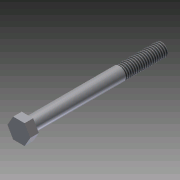
# Autodesk Inventor part: Bolt 1764
Saved by Autodesk Inventor 2011 (Build 150239000, 239)
## iProperties
Created: 2010-02-11
Part Number: Bolt 1764
Document SubType Name: Modeling
Designer: jrobinson
Density: 1 g/cm^3
Author: jrobinson
Autodesk Inventor part; units mm, degrees
ref_plane "YZ Plane" through (0, 0, 0) normal (1, 0, 0) x (0, 1, 0)
ref_plane "XZ Plane" through (0, 0, 0) normal (0, 1, 0) x (-1, 0, 0)
ref_plane "XY Plane" through (0, 0, 0) normal (0, 0, 1) x (1, 0, 0)
sketch "Sketch1" plane through (0, 0, 0) normal (0, 0, 1) x (1, 0, 0)
  circle A0 centre (0, 0) radius 4.6609
  dimension "d0" = 9.3218
  constraints: 1 centre point, 1 coincident
  measures "d0" diameter of A0
extrude "Extrusion1" add sketch "Sketch1" along normal blind 94.996
thread "Thread1" size "3/8-16 UNC" class "2A" standard "ANSI Unified Screw Threads" length 29.845
sketch "Sketch2" plane through (0, 0, 94.996) normal (0, 0, 1) x (1, 0, 0)
  circle A0 centre (0, 0) radius 4.6609 projected
  line L0 (8.0949, 0) -> (4.0475, -7.0104)
  line L1 (4.0475, -7.0104) -> (-4.0475, -7.0104)
  line L2 (-4.0475, -7.0104) -> (-8.0949, 0)
  line L3 (-8.0949, 0) -> (-4.0475, 7.0104)
  line L4 (-4.0475, 7.0104) -> (4.0475, 7.0104)
  line L5 (4.0475, 7.0104) -> (8.0949, 0)
  dimension "d5" = 14.0208
  constraints: 12 end point, 1 coincident, 13 other
  measures "d5" distance between parallel lines of L4 L1
extrude "Extrusion2" add sketch "Sketch2" along normal blind 6.0706 contours A0 | L0 L1 L2 L3 L4 L5
body "Solid1"
